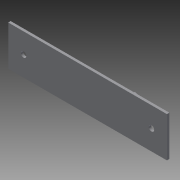
# Autodesk Inventor part: tabliczka tworcy i opiekun boki skrzynki
Saved by Autodesk Inventor 2014 (Build 180170000, 170)
## iProperties
Created: 2018-03-23
Part Number: tabliczka tworcy i opiekun boki skrzynki
Material: Generic
Document SubType Name: Modeling
Designer: HP820
Density: 1 g/cm^3
Appearance: Default
Author: HP820
Autodesk Inventor part; units mm, degrees
(part 1 of 3)
ref_plane "YZ Plane" through (0, 0, 0) normal (1, 0, 0) x (0, 1, 0)
ref_plane "XZ Plane" through (0, 0, 0) normal (0, 1, 0) x (-1, 0, 0)
ref_plane "XY Plane" through (0, 0, 0) normal (0, 0, 1) x (1, 0, 0)
sketch "Sketch1" plane through (0, 0, 0) normal (0, 1, 0) x (-1, 0, 0)
  line L0 (-51.5, 13) -> (51.5, 13)
  line L1 (51.5, 13) -> (51.5, -13)
  line L2 (51.5, -13) -> (-51.5, -13)
  line L3 (-51.5, -13) -> (-51.5, 13)
  line L4 (-51.5, 13) -> (51.5, -13) construction
  line L5 (51.5, 13) -> (-51.5, -13) construction
  point P0 (0, 0)
  dimension "d0" = 103
  dimension "d1" = 26
  constraints: 12 end point, 2 midpoint, 2 parallel, 1 horizontal, 1 perpendicular
  measures "d0" distance of L1.end L2.end
  measures "d1" distance of L0.end L1.end
extrude "Extrusion1" add sketch "Sketch1" along normal blind 1.6
sketch "Sketch2" plane through (0, 1.6, 0) normal (0, 1, 0) x (1, 0, 0)
  line L0 (-48.6354, 11.3005) -> (49.671, 11.3005) construction
  line L1 (49.671, 11.3005) -> (49.671, -11.1656) construction
  line L2 (49.671, -11.1656) -> (-48.6354, -11.1656) construction
  line L3 (-48.6354, -11.1656) -> (-48.6354, 11.3005) construction
  spline S0 degree 2 poles (-15.1532, 10.858) (-15.1532, 10.6489) (-15.2869, 10.2696) (-15.4109, 10.1432) knots 0 0 0 1 2 2 2
  spline S1 degree 2 poles (-15.4109, 10.1432) (-15.4863, 10.063) (-15.671, 9.9317) (-15.7804, 9.8855) knots 0 0 0 1 2 2 2
  spline S2 degree 2 poles (-15.7804, 9.8855) (-15.8923, 9.8393) (-16.1524, 9.7858) (-16.3128, 9.7858) knots 0 0 0 1 2 2 2
  line L4 (-16.3128, 9.7858) -> (-16.7067, 9.7858)
  line L5 (-16.7067, 9.7858) -> (-16.7067, 8.8037)
  line L6 (-16.7067, 8.8037) -> (-17.4603, 8.8037)
  line L7 (-17.4603, 8.8037) -> (-17.4603, 11.8037)
  line L8 (-17.4603, 11.8037) -> (-16.2958, 11.8037)
  spline S3 degree 2 poles (-16.2958, 11.8037) (-16.0381, 11.8037) (-15.6613, 11.7089) (-15.5081, 11.6068) knots 0 0 0 1 2 2 2
  spline S4 degree 2 poles (-15.5081, 11.6068) (-15.338, 11.4925) (-15.1532, 11.1181) (-15.1532, 10.858) knots 0 0 0 1 2 2 2
  spline S5 degree 2 poles (-15.9263, 10.8385) (-15.9263, 10.9674) (-16.0479, 11.1497) (-16.1305, 11.1837) knots 0 0 0 1 2 2 2
  spline S6 degree 2 poles (-16.1305, 11.1837) (-16.2375, 11.2299) (-16.432, 11.2445) (-16.5997, 11.2445) knots 0 0 0 1 2 2 2
  line L9 (-16.5997, 11.2445) -> (-16.7067, 11.2445)
  line L10 (-16.7067, 11.2445) -> (-16.7067, 10.345)
  line L11 (-16.7067, 10.345) -> (-16.6532, 10.345)
  spline S7 degree 2 poles (-16.6532, 10.345) (-16.5487, 10.345) (-16.359, 10.3499) (-16.2885, 10.362) knots 0 0 0 1 2 2 2
  spline S8 degree 2 poles (-16.2885, 10.362) (-16.2278, 10.3717) (-16.094, 10.4301) (-16.0576, 10.4666) knots 0 0 0 1 2 2 2
  spline S9 degree 2 poles (-16.0576, 10.4666) (-15.9798, 10.5395) (-15.9263, 10.7024) (-15.9263, 10.8385) knots 0 0 0 1 2 2 2
  line L12 (-13.2715, 10.3985) -> (-13.3299, 10.3985)
  spline S10 degree 2 poles (-13.3299, 10.3985) (-13.3712, 10.4131) (-13.5244, 10.4277) (-13.6167, 10.4277) knots 0 0 0 1 2 2 2
  spline S11 degree 2 poles (-13.6167, 10.4277) (-13.7261, 10.4277) (-13.9717, 10.362) (-14.0859, 10.3183) knots 0 0 0 1 2 2 2
  line L13 (-14.0859, 10.3183) -> (-14.0859, 8.8037)
  line L14 (-14.0859, 8.8037) -> (-14.791, 8.8037)
  line L15 (-14.791, 8.8037) -> (-14.791, 11.067)
  line L16 (-14.791, 11.067) -> (-14.0859, 11.067)
  line L17 (-14.0859, 11.067) -> (-14.0859, 10.7413)
  spline S12 degree 2 poles (-14.0859, 10.7413) (-14.0373, 10.785) (-13.8671, 10.9212) (-13.7966, 10.9625) knots 0 0 0 1 2 2 2
  spline S13 degree 2 poles (-13.7966, 10.9625) (-13.7188, 11.0087) (-13.5146, 11.0743) (-13.4247, 11.0743) knots 0 0 0 1 2 2 2
  spline S14 degree 2 poles (-13.4247, 11.0743) (-13.3906, 11.0743) (-13.3056, 11.0695) (-13.2715, 11.067) knots 0 0 0 1 2 2 2
  line L18 (-13.2715, 11.067) -> (-13.2715, 10.3985)
  spline S15 degree 2 poles (-10.8307, 9.9341) (-10.8307, 9.375) (-11.4409, 8.7332) (-11.9976, 8.7332) knots 0 0 0 1 2 2 2
  spline S16 degree 2 poles (-11.9976, 8.7332) (-12.5519, 8.7332) (-13.167, 9.375) (-13.167, 9.9341) knots 0 0 0 1 2 2 2
  spline S17 degree 2 poles (-13.167, 9.9341) (-13.167, 10.4982) (-12.5519, 11.1376) (-11.9976, 11.1376) knots 0 0 0 1 2 2 2
  spline S18 degree 2 poles (-11.9976, 11.1376) (-11.4433, 11.1376) (-10.8307, 10.4957) (-10.8307, 9.9341) knots 0 0 0 1 2 2 2
  spline S19 degree 2 poles (-11.5527, 9.9293) (-11.5527, 10.1311) (-11.6184, 10.4009) (-11.6767, 10.4811) knots 0 0 0 1 2 2 2
  spline S20 degree 2 poles (-11.6767, 10.4811) (-11.7399, 10.5662) (-11.8979, 10.6319) (-11.9976, 10.6319) knots 0 0 0 1 2 2 2
  spline S21 degree 2 poles (-11.9976, 10.6319) (-12.0949, 10.6319) (-12.248, 10.5735) (-12.3112, 10.4909) knots 0 0 0 1 2 2 2
  spline S22 degree 2 poles (-12.3112, 10.4909) (-12.372, 10.4131) (-12.4449, 10.1384) (-12.4449, 9.9293) knots 0 0 0 1 2 2 2
  spline S23 degree 2 poles (-12.4449, 9.9293) (-12.4449, 9.7226) (-12.3769, 9.4674) (-12.321, 9.3896) knots 0 0 0 1 2 2 2
  spline S24 degree 2 poles (-12.321, 9.3896) (-12.265, 9.3118) (-12.0949, 9.2388) (-11.9927, 9.2388) knots 0 0 0 1 2 2 2
  spline S25 degree 2 poles (-11.9927, 9.2388) (-11.9077, 9.2388) (-11.7326, 9.3118) (-11.6791, 9.3847) knots 0 0 0 1 2 2 2
  spline S26 degree 2 poles (-11.6791, 9.3847) (-11.6184, 9.4698) (-11.5527, 9.7153) (-11.5527, 9.9293) knots 0 0 0 1 2 2 2
  spline S27 degree 2 poles (-9.4984, 8.7648) (-9.4984, 8.3807) (-9.953, 7.9528) (-10.3128, 7.9528) knots 0 0 0 1 2 2 2
  spline S28 degree 2 poles (-10.3128, 7.9528) (-10.5073, 7.9528) (-10.821, 7.9868) (-10.8939, 8.0063) knots 0 0 0 1 2 2 2
  line L19 (-10.8939, 8.0063) -> (-10.8939, 8.5265)
  line L20 (-10.8939, 8.5265) -> (-10.8404, 8.5265)
  spline S29 degree 2 poles (-10.8404, 8.5265) (-10.7699, 8.5047) (-10.6046, 8.4779) (-10.5535, 8.4779) knots 0 0 0 1 2 2 2
  spline S30 degree 2 poles (-10.5535, 8.4779) (-10.3493, 8.4779) (-10.2034, 8.7283) (-10.2034, 9.0128) knots 0 0 0 1 2 2 2
  line L21 (-10.2034, 9.0128) -> (-10.2034, 10.576)
  line L22 (-10.2034, 10.576) -> (-10.6094, 10.576)
  line L23 (-10.6094, 10.576) -> (-10.6094, 11.067)
  line L24 (-10.6094, 11.067) -> (-9.4984, 11.067)
  line L25 (-9.4984, 11.067) -> (-9.4984, 8.7648)
  line L26 (-9.4984, 11.3904) -> (-10.2496, 11.3904)
  line L27 (-10.2496, 11.3904) -> (-10.2496, 11.9398)
  line L28 (-10.2496, 11.9398) -> (-9.4984, 11.9398)
  line L29 (-9.4984, 11.9398) -> (-9.4984, 11.3904)
  spline S31 degree 2 poles (-7.7991, 8.7429) (-8.4409, 8.7429) (-9.124, 9.3555) (-9.124, 9.922) knots 0 0 0 1 2 2 2
  spline S32 degree 2 poles (-9.124, 9.922) (-9.124, 10.4763) (-8.4871, 11.1376) (-7.9133, 11.1376) knots 0 0 0 1 2 2 2
  spline S33 degree 2 poles (-7.9133, 11.1376) (-7.3955, 11.1376) (-6.8704, 10.576) (-6.8704, 10.0557) knots 0 0 0 1 2 2 2
  line L30 (-6.8704, 10.0557) -> (-6.8704, 9.8004)
  line L31 (-6.8704, 9.8004) -> (-8.419, 9.8004)
  spline S34 degree 2 poles (-8.419, 9.8004) (-8.4093, 9.6424) (-8.295, 9.4333) (-8.2026, 9.3701) knots 0 0 0 1 2 2 2
  spline S35 degree 2 poles (-8.2026, 9.3701) (-8.1127, 9.3069) (-7.8696, 9.2534) (-7.7261, 9.2534) knots 0 0 0 1 2 2 2
  spline S36 degree 2 poles (-7.7261, 9.2534) (-7.6046, 9.2534) (-7.3663, 9.3069) (-7.2667, 9.3531) knots 0 0 0 1 2 2 2
  spline S37 degree 2 poles (-7.2667, 9.3531) (-7.1791, 9.3896) (-7.0333, 9.4795) (-6.9871, 9.5136) knots 0 0 0 1 2 2 2
  line L32 (-6.9871, 9.5136) -> (-6.9117, 9.5136)
  line L33 (-6.9117, 9.5136) -> (-6.9117, 8.9301)
  spline S38 degree 2 poles (-6.9117, 8.9301) (-6.9992, 8.8961) (-7.1402, 8.8377) (-7.2667, 8.8085) knots 0 0 0 1 2 2 2
  spline S39 degree 2 poles (-7.2667, 8.8085) (-7.3809, 8.7769) (-7.624, 8.7429) (-7.7991, 8.7429) knots 0 0 0 1 2 2 2
  spline S40 degree 2 poles (-7.5657, 10.2259) (-7.5705, 10.4495) (-7.7675, 10.6854) (-7.9692, 10.6854) knots 0 0 0 1 2 2 2
  spline S41 degree 2 poles (-7.9692, 10.6854) (-8.1759, 10.6854) (-8.4093, 10.4374) (-8.4214, 10.2259) knots 0 0 0 1 2 2 2
  line L34 (-8.4214, 10.2259) -> (-7.5657, 10.2259)
  line L35 (-4.2423, 8.8037) -> (-5.0811, 8.8037)
  line L36 (-5.0811, 8.8037) -> (-5.6937, 9.7858)
  line L37 (-5.6937, 9.7858) -> (-5.8031, 9.64)
  line L38 (-5.8031, 9.64) -> (-5.8031, 8.8037)
  line L39 (-5.8031, 8.8037) -> (-6.5081, 8.8037)
  line L40 (-6.5081, 8.8037) -> (-6.5081, 11.9374)
  line L41 (-6.5081, 11.9374) -> (-5.8031, 11.9374)
  line L42 (-5.8031, 11.9374) -> (-5.8031, 10.1821)
  line L43 (-5.8031, 10.1821) -> (-5.1346, 11.067)
  line L44 (-5.1346, 11.067) -> (-4.3007, 11.067)
  line L45 (-4.3007, 11.067) -> (-5.0932, 10.0922)
  line L46 (-5.0932, 10.0922) -> (-4.2423, 8.8037)
  spline S42 degree 2 poles (-3.1556, 8.7599) (-3.5859, 8.7599) (-3.9798, 9.1149) (-3.9798, 9.5184) knots 0 0 0 1 2 2 2
  line L47 (-3.9798, 9.5184) -> (-3.9798, 10.576)
  line L48 (-3.9798, 10.576) -> (-4.2496, 10.576)
  line L49 (-4.2496, 10.576) -> (-4.2496, 11.067)
  line L50 (-4.2496, 11.067) -> (-3.9798, 11.067)
  line L51 (-3.9798, 11.067) -> (-3.9798, 11.7137)
  line L52 (-3.9798, 11.7137) -> (-3.2748, 11.7137)
  line L53 (-3.2748, 11.7137) -> (-3.2748, 11.067)
  line L54 (-3.2748, 11.067) -> (-2.594, 11.067)
  line L55 (-2.594, 11.067) -> (-2.594, 10.576)
  line L56 (-2.594, 10.576) -> (-3.2748, 10.576)
  line L57 (-3.2748, 10.576) -> (-3.2748, 9.7713)
  spline S43 degree 2 poles (-3.2748, 9.7713) (-3.2748, 9.6521) (-3.2699, 9.4747) (-3.2407, 9.4042) knots 0 0 0 1 2 2 2
  spline S44 degree 2 poles (-3.2407, 9.4042) (-3.2115, 9.3337) (-3.0681, 9.251) (-2.932, 9.251) knots 0 0 0 1 2 2 2
  spline S45 degree 2 poles (-2.932, 9.251) (-2.8736, 9.251) (-2.6913, 9.2996) (-2.6548, 9.3191) knots 0 0 0 1 2 2 2
  line L58 (-2.6548, 9.3191) -> (-2.594, 9.3191)
  line L59 (-2.594, 9.3191) -> (-2.594, 8.8231)
  spline S46 degree 2 poles (-2.594, 8.8231) (-2.7083, 8.794) (-2.966, 8.7599) (-3.1556, 8.7599) knots 0 0 0 1 2 2 2
  line L60 (2.2731, 11.067) -> (1.6118, 8.8037)
  line L61 (1.6118, 8.8037) -> (0.863, 8.8037)
  line L62 (0.863, 8.8037) -> (0.4643, 10.2672)
  line L63 (0.4643, 10.2672) -> (0.0656, 8.8037)
  line L64 (0.0656, 8.8037) -> (-0.6832, 8.8037)
  line L65 (-0.6832, 8.8037) -> (-1.3396, 11.067)
  line L66 (-1.3396, 11.067) -> (-0.5981, 11.067)
  line L67 (-0.5981, 11.067) -> (-0.2504, 9.5695)
  line L68 (-0.2504, 9.5695) -> (0.1774, 11.067)
  line L69 (0.1774, 11.067) -> (0.8022, 11.067)
  line L70 (0.8022, 11.067) -> (1.2058, 9.5695)
  line L71 (1.2058, 9.5695) -> (1.5486, 11.067)
  line L72 (1.5486, 11.067) -> (2.2731, 11.067)
  line L73 (4.6823, 11.067) -> (3.5421, 7.9747)
  line L74 (3.5421, 7.9747) -> (2.7836, 7.9747)
  line L75 (2.7836, 7.9747) -> (3.1264, 8.8596)
  line L76 (3.1264, 8.8596) -> (2.2974, 11.067)
  line L77 (2.2974, 11.067) -> (3.0364, 11.067)
  line L78 (3.0364, 11.067) -> (3.5129, 9.6473)
  line L79 (3.5129, 9.6473) -> (3.9578, 11.067)
  line L80 (3.9578, 11.067) -> (4.6823, 11.067)
  line L81 (7.2131, 8.8037) -> (6.3744, 8.8037)
  line L82 (6.3744, 8.8037) -> (5.7617, 9.7858)
  line L83 (5.7617, 9.7858) -> (5.6523, 9.64)
  line L84 (5.6523, 9.64) -> (5.6523, 8.8037)
  line L85 (5.6523, 8.8037) -> (4.9473, 8.8037)
  line L86 (4.9473, 8.8037) -> (4.9473, 11.9374)
  line L87 (4.9473, 11.9374) -> (5.6523, 11.9374)
  line L88 (5.6523, 11.9374) -> (5.6523, 10.1821)
  line L89 (5.6523, 10.1821) -> (6.3209, 11.067)
  line L90 (6.3209, 11.067) -> (7.1547, 11.067)
  line L91 (7.1547, 11.067) -> (6.3622, 10.0922)
  line L92 (6.3622, 10.0922) -> (7.2131, 8.8037)
  spline S47 degree 2 poles (9.6053, 9.9341) (9.6053, 9.375) (8.9951, 8.7332) (8.4384, 8.7332) knots 0 0 0 1 2 2 2
  spline S48 degree 2 poles (8.4384, 8.7332) (7.8841, 8.7332) (7.269, 9.375) (7.269, 9.9341) knots 0 0 0 1 2 2 2
  spline S49 degree 2 poles (7.269, 9.9341) (7.269, 10.4982) (7.8841, 11.1376) (8.4384, 11.1376) knots 0 0 0 1 2 2 2
  spline S50 degree 2 poles (8.4384, 11.1376) (8.9927, 11.1376) (9.6053, 10.4957) (9.6053, 9.9341) knots 0 0 0 1 2 2 2
  spline S51 degree 2 poles (8.8833, 9.9293) (8.8833, 10.1311) (8.8176, 10.4009) (8.7593, 10.4811) knots 0 0 0 1 2 2 2
  spline S52 degree 2 poles (8.7593, 10.4811) (8.6961, 10.5662) (8.538, 10.6319) (8.4384, 10.6319) knots 0 0 0 1 2 2 2
  spline S53 degree 2 poles (8.4384, 10.6319) (8.3411, 10.6319) (8.188, 10.5735) (8.1248, 10.4909) knots 0 0 0 1 2 2 2
  spline S54 degree 2 poles (8.1248, 10.4909) (8.064, 10.4131) (7.991, 10.1384) (7.991, 9.9293) knots 0 0 0 1 2 2 2
  spline S55 degree 2 poles (7.991, 9.9293) (7.991, 9.7226) (8.0591, 9.4674) (8.115, 9.3896) knots 0 0 0 1 2 2 2
  spline S56 degree 2 poles (8.115, 9.3896) (8.1709, 9.3118) (8.3411, 9.2388) (8.4432, 9.2388) knots 0 0 0 1 2 2 2
  spline S57 degree 2 poles (8.4432, 9.2388) (8.5283, 9.2388) (8.7034, 9.3118) (8.7568, 9.3847) knots 0 0 0 1 2 2 2
  spline S58 degree 2 poles (8.7568, 9.3847) (8.8176, 9.4698) (8.8833, 9.7153) (8.8833, 9.9293) knots 0 0 0 1 2 2 2
  line L93 (12.0972, 8.8037) -> (11.3873, 8.8037)
  line L94 (11.3873, 8.8037) -> (11.3873, 9.9244)
  spline S59 degree 2 poles (11.3873, 9.9244) (11.3873, 10.063) (11.3654, 10.3353) (11.3363, 10.3985) knots 0 0 0 1 2 2 2
  spline S60 degree 2 poles (11.3363, 10.3985) (11.2998, 10.4763) (11.1637, 10.5419) (11.047, 10.5419) knots 0 0 0 1 2 2 2
  spline S61 degree 2 poles (11.047, 10.5419) (10.9619, 10.5419) (10.7844, 10.4763) (10.6847, 10.4058) knots 0 0 0 1 2 2 2
  line L95 (10.6847, 10.4058) -> (10.6847, 8.8037)
  line L96 (10.6847, 8.8037) -> (9.9797, 8.8037)
  line L97 (9.9797, 8.8037) -> (9.9797, 11.067)
  line L98 (9.9797, 11.067) -> (10.6847, 11.067)
  line L99 (10.6847, 11.067) -> (10.6847, 10.8166)
  spline S62 degree 2 poles (10.6847, 10.8166) (10.8573, 10.9625) (11.1855, 11.1278) (11.3849, 11.1278) knots 0 0 0 1 2 2 2
  spline S63 degree 2 poles (11.3849, 11.1278) (11.7301, 11.1278) (12.0972, 10.6902) (12.0972, 10.2769) knots 0 0 0 1 2 2 2
  line L100 (12.0972, 10.2769) -> (12.0972, 8.8037)
  spline S64 degree 2 poles (13.8671, 9.0444) (13.7941, 8.9836) (13.6799, 8.8863) (13.5826, 8.8377) knots 0 0 0 1 2 2 2
  spline S65 degree 2 poles (13.5826, 8.8377) (13.4878, 8.7915) (13.3079, 8.7429) (13.1474, 8.7429) knots 0 0 0 1 2 2 2
  spline S66 degree 2 poles (13.1474, 8.7429) (12.846, 8.7429) (12.4497, 9.1465) (12.4497, 9.4528) knots 0 0 0 1 2 2 2
  spline S67 degree 2 poles (12.4497, 9.4528) (12.4497, 9.7032) (12.6515, 10.0144) (12.8411, 10.1043) knots 0 0 0 1 2 2 2
  spline S68 degree 2 poles (12.8411, 10.1043) (13.0332, 10.1967) (13.5656, 10.2696) (13.8719, 10.2891) knots 0 0 0 1 2 2 2
  line L101 (13.8719, 10.2891) -> (13.8719, 10.3012)
  spline S69 degree 2 poles (13.8719, 10.3012) (13.8719, 10.4884) (13.5948, 10.6319) (13.3176, 10.6319) knots 0 0 0 1 2 2 2
  spline S70 degree 2 poles (13.3176, 10.6319) (13.1936, 10.6319) (12.8581, 10.5419) (12.7001, 10.4714) knots 0 0 0 1 2 2 2
  line L102 (12.7001, 10.4714) -> (12.6393, 10.4714)
  line L103 (12.6393, 10.4714) -> (12.6393, 11.0184)
  spline S71 degree 2 poles (12.6393, 11.0184) (12.7439, 11.0476) (13.2107, 11.1303) (13.4489, 11.1303) knots 0 0 0 1 2 2 2
  spline S72 degree 2 poles (13.4489, 11.1303) (14.0324, 11.1303) (14.5672, 10.7413) (14.5672, 10.3426) knots 0 0 0 1 2 2 2
  line L104 (14.5672, 10.3426) -> (14.5672, 8.8037)
  line L105 (14.5672, 8.8037) -> (13.8671, 8.8037)
  line L106 (13.8671, 8.8037) -> (13.8671, 9.0444)
  line L107 (13.8671, 9.3944) -> (13.8671, 9.8636)
  spline S73 degree 2 poles (13.8671, 9.8636) (13.6872, 9.8466) (13.4659, 9.8199) (13.359, 9.781) knots 0 0 0 1 2 2 2
  spline S74 degree 2 poles (13.359, 9.781) (13.2641, 9.7494) (13.162, 9.6181) (13.162, 9.5111) knots 0 0 0 1 2 2 2
  spline S75 degree 2 poles (13.162, 9.5111) (13.162, 9.3531) (13.3346, 9.234) (13.5024, 9.234) knots 0 0 0 1 2 2 2
  spline S76 degree 2 poles (13.5024, 9.234) (13.5948, 9.234) (13.7893, 9.3191) (13.8671, 9.3944) knots 0 0 0 1 2 2 2
  line L108 (15.7949, 8.8037) -> (15.0899, 8.8037)
  line L109 (15.0899, 8.8037) -> (15.0899, 11.9374)
  line L110 (15.0899, 11.9374) -> (15.7949, 11.9374)
  line L111 (15.7949, 11.9374) -> (15.7949, 8.8037)
  line L112 (17.0397, 8.8037) -> (16.3346, 8.8037)
  line L113 (16.3346, 8.8037) -> (16.3346, 11.067)
  line L114 (16.3346, 11.067) -> (17.0397, 11.067)
  line L115 (17.0397, 11.067) -> (17.0397, 8.8037)
  line L116 (17.0615, 11.3904) -> (16.3152, 11.3904)
  line L117 (16.3152, 11.3904) -> (16.3152, 11.9398)
  line L118 (16.3152, 11.9398) -> (17.0615, 11.9398)
  line L119 (17.0615, 11.9398) -> (17.0615, 11.3904)
  line L120 (18.4157, 8.8037) -> (17.7034, 8.8037)
  line L121 (17.7034, 8.8037) -> (17.7034, 9.5962)
  line L122 (17.7034, 9.5962) -> (18.4157, 9.5962)
  line L123 (18.4157, 9.5962) -> (18.4157, 8.8037)
  line L124 (18.4157, 10.2745) -> (17.7034, 10.2745)
  line L125 (17.7034, 10.2745) -> (17.7034, 11.067)
  line L126 (17.7034, 11.067) -> (18.4157, 11.067)
  line L127 (18.4157, 11.067) -> (18.4157, 10.2745)
  line L128 (-19.4137, 3.8643) -> (-21.4145, 3.8643)
  line L129 (-21.4145, 3.8643) -> (-21.4145, 4.8173)
  line L130 (-21.4145, 4.8173) -> (-21.7573, 4.613)
  line L131 (-21.7573, 4.613) -> (-21.7573, 5.0968)
  line L132 (-21.7573, 5.0968) -> (-21.4145, 5.2962)
  line L133 (-21.4145, 5.2962) -> (-21.4145, 6.8643)
  line L134 (-21.4145, 6.8643) -> (-20.6658, 6.8643)
  line L135 (-20.6658, 6.8643) -> (-20.6658, 5.7095)
  line L136 (-20.6658, 5.7095) -> (-20.0191, 6.096)
  line L137 (-20.0191, 6.096) -> (-20.0191, 5.6122)
  line L138 (-20.0191, 5.6122) -> (-20.6658, 5.2305)
  line L139 (-20.6658, 5.2305) -> (-20.6658, 4.4356)
  line L140 (-20.6658, 4.4356) -> (-19.4137, 4.4356)
  line L141 (-19.4137, 4.4356) -> (-19.4137, 3.8643)
  line L142 (-16.9948, 3.8643) -> (-17.6998, 3.8643)
  line L143 (-17.6998, 3.8643) -> (-17.6998, 4.1147)
  spline S77 degree 2 poles (-17.6998, 4.1147) (-17.8821, 3.9615) (-18.1885, 3.801) (-18.4, 3.801) knots 0 0 0 1 2 2 2
  spline S78 degree 2 poles (-18.4, 3.801) (-18.7355, 3.801) (-19.1123, 4.2265) (-19.1123, 4.6544) knots 0 0 0 1 2 2 2
  line L144 (-19.1123, 4.6544) -> (-19.1123, 6.1276)
  line L145 (-19.1123, 6.1276) -> (-18.4024, 6.1276)
  line L146 (-18.4024, 6.1276) -> (-18.4024, 5.0045)
  spline S79 degree 2 poles (-18.4024, 5.0045) (-18.4024, 4.8294) (-18.3854, 4.6057) (-18.3513, 4.5304) knots 0 0 0 1 2 2 2
  spline S80 degree 2 poles (-18.3513, 4.5304) (-18.3173, 4.4599) (-18.1836, 4.3869) (-18.062, 4.3869) knots 0 0 0 1 2 2 2
  spline S81 degree 2 poles (-18.062, 4.3869) (-17.9891, 4.3869) (-17.7849, 4.4599) (-17.6998, 4.5231) knots 0 0 0 1 2 2 2
  line L147 (-17.6998, 4.5231) -> (-17.6998, 6.1276)
  line L148 (-17.6998, 6.1276) -> (-16.9948, 6.1276)
  line L149 (-16.9948, 6.1276) -> (-16.9948, 3.8643)
  line L150 (-14.1893, 3.8643) -> (-15.028, 3.8643)
  line L151 (-15.028, 3.8643) -> (-15.6406, 4.8464)
  line L152 (-15.6406, 4.8464) -> (-15.75, 4.7006)
  line L153 (-15.75, 4.7006) -> (-15.75, 3.8643)
  line L154 (-15.75, 3.8643) -> (-16.4551, 3.8643)
  line L155 (-16.4551, 3.8643) -> (-16.4551, 6.998)
  line L156 (-16.4551, 6.998) -> (-15.75, 6.998)
  line L157 (-15.75, 6.998) -> (-15.75, 5.2427)
  line L158 (-15.75, 5.2427) -> (-15.0815, 6.1276)
  line L159 (-15.0815, 6.1276) -> (-14.2476, 6.1276)
  line L160 (-14.2476, 6.1276) -> (-15.0402, 5.1527)
  line L161 (-15.0402, 5.1527) -> (-14.1893, 3.8643)
  spline S82 degree 2 poles (-12.7209, 4.1049) (-12.7938, 4.0442) (-12.9081, 3.9469) (-13.0053, 3.8983) knots 0 0 0 1 2 2 2
  spline S83 degree 2 poles (-13.0053, 3.8983) (-13.1001, 3.8521) (-13.28, 3.8035) (-13.4405, 3.8035) knots 0 0 0 1 2 2 2
  spline S84 degree 2 poles (-13.4405, 3.8035) (-13.7419, 3.8035) (-14.1382, 4.207) (-14.1382, 4.5134) knots 0 0 0 1 2 2 2
  spline S85 degree 2 poles (-14.1382, 4.5134) (-14.1382, 4.7638) (-13.9364, 5.075) (-13.7468, 5.1649) knots 0 0 0 1 2 2 2
  spline S86 degree 2 poles (-13.7468, 5.1649) (-13.5547, 5.2573) (-13.0223, 5.3302) (-12.716, 5.3497) knots 0 0 0 1 2 2 2
  line L162 (-12.716, 5.3497) -> (-12.716, 5.3618)
  spline S87 degree 2 poles (-12.716, 5.3618) (-12.716, 5.549) (-12.9932, 5.6925) (-13.2703, 5.6925) knots 0 0 0 1 2 2 2
  spline S88 degree 2 poles (-13.2703, 5.6925) (-13.3943, 5.6925) (-13.7298, 5.6025) (-13.8878, 5.532) knots 0 0 0 1 2 2 2
  line L163 (-13.8878, 5.532) -> (-13.9486, 5.532)
  line L164 (-13.9486, 5.532) -> (-13.9486, 6.079)
  spline S89 degree 2 poles (-13.9486, 6.079) (-13.844, 6.1082) (-13.3773, 6.1908) (-13.139, 6.1908) knots 0 0 0 1 2 2 2
  spline S90 degree 2 poles (-13.139, 6.1908) (-12.5556, 6.1908) (-12.0207, 5.8019) (-12.0207, 5.4032) knots 0 0 0 1 2 2 2
  line L165 (-12.0207, 5.4032) -> (-12.0207, 3.8643)
  line L166 (-12.0207, 3.8643) -> (-12.7209, 3.8643)
  line L167 (-12.7209, 3.8643) -> (-12.7209, 4.1049)
  line L168 (-12.7209, 4.455) -> (-12.7209, 4.9242)
  spline S91 degree 2 poles (-12.7209, 4.9242) (-12.9008, 4.9072) (-13.122, 4.8805) (-13.229, 4.8416) knots 0 0 0 1 2 2 2
  spline S92 degree 2 poles (-13.229, 4.8416) (-13.3238, 4.81) (-13.4259, 4.6787) (-13.4259, 4.5717) knots 0 0 0 1 2 2 2
  spline S93 degree 2 poles (-13.4259, 4.5717) (-13.4259, 4.4137) (-13.2533, 4.2946) (-13.0855, 4.2946) knots 0 0 0 1 2 2 2
  spline S94 degree 2 poles (-13.0855, 4.2946) (-12.9932, 4.2946) (-12.7987, 4.3797) (-12.7209, 4.455) knots 0 0 0 1 2 2 2
  spline S95 degree 2 poles (-10.81, 3.8035) (-11.058, 3.8035) (-11.5029, 3.9129) (-11.6487, 3.9858) knots 0 0 0 1 2 2 2
  line L169 (-11.6487, 3.9858) -> (-11.6487, 4.5814)
  line L170 (-11.6487, 4.5814) -> (-11.5904, 4.5814)
  spline S96 degree 2 poles (-11.5904, 4.5814) (-11.5393, 4.5425) (-11.4105, 4.4502) (-11.2962, 4.3991) knots 0 0 0 1 2 2 2
  spline S97 degree 2 poles (-11.2962, 4.3991) (-11.1966, 4.3529) (-10.951, 4.2873) (-10.8051, 4.2873) knots 0 0 0 1 2 2 2
  spline S98 degree 2 poles (-10.8051, 4.2873) (-10.6569, 4.2873) (-10.4283, 4.3797) (-10.4283, 4.4793) knots 0 0 0 1 2 2 2
  spline S99 degree 2 poles (-10.4283, 4.4793) (-10.4283, 4.5571) (-10.5329, 4.6398) (-10.6836, 4.6738) knots 0 0 0 1 2 2 2
  spline S100 degree 2 poles (-10.6836, 4.6738) (-10.7638, 4.6957) (-11.0094, 4.7419) (-11.1042, 4.7711) knots 0 0 0 1 2 2 2
  spline S101 degree 2 poles (-11.1042, 4.7711) (-11.3716, 4.8537) (-11.639, 5.1771) (-11.639, 5.4421) knots 0 0 0 1 2 2 2
  spline S102 degree 2 poles (-11.639, 5.4421) (-11.639, 5.5928) (-11.5004, 5.8602) (-11.3643, 5.9647) knots 0 0 0 1 2 2 2
  spline S103 degree 2 poles (-11.3643, 5.9647) (-11.2306, 6.0669) (-10.8343, 6.1884) (-10.5839, 6.1884) knots 0 0 0 1 2 2 2
  spline S104 degree 2 poles (-10.5839, 6.1884) (-10.3457, 6.1884) (-9.947, 6.0936) (-9.8108, 6.028) knots 0 0 0 1 2 2 2
  line L171 (-9.8108, 6.028) -> (-9.8108, 5.4542)
  line L172 (-9.8108, 5.4542) -> (-9.8667, 5.4542)
  spline S105 degree 2 poles (-9.8667, 5.4542) (-9.9032, 5.4834) (-10.0612, 5.5782) (-10.1342, 5.6122) knots 0 0 0 1 2 2 2
  spline S106 degree 2 poles (-10.1342, 5.6122) (-10.2241, 5.6511) (-10.4429, 5.7046) (-10.5572, 5.7046) knots 0 0 0 1 2 2 2
  spline S107 degree 2 poles (-10.5572, 5.7046) (-10.7103, 5.7046) (-10.9218, 5.6001) (-10.9218, 5.515) knots 0 0 0 1 2 2 2
  spline S108 degree 2 poles (-10.9218, 5.515) (-10.9218, 5.4372) (-10.8173, 5.3497) (-10.6423, 5.3059) knots 0 0 0 1 2 2 2
  spline S109 degree 2 poles (-10.6423, 5.3059) (-10.5523, 5.284) (-10.3165, 5.2427) (-10.2071, 5.2062) knots 0 0 0 1 2 2 2
  spline S110 degree 2 poles (-10.2071, 5.2062) (-9.964, 5.1284) (-9.7111, 4.8245) (-9.7111, 4.5717) knots 0 0 0 1 2 2 2
  spline S111 degree 2 poles (-9.7111, 4.5717) (-9.7111, 4.4137) (-9.8594, 4.1244) (-9.998, 4.0271) knots 0 0 0 1 2 2 2
  spline S112 degree 2 poles (-9.998, 4.0271) (-10.1415, 3.9202) (-10.5353, 3.8035) (-10.81, 3.8035) knots 0 0 0 1 2 2 2
  line L173 (-7.5718, 3.8643) -> (-9.5483, 3.8643)
  line L174 (-9.5483, 3.8643) -> (-9.5483, 4.3286)
  line L175 (-9.5483, 4.3286) -> (-8.4688, 5.5976)
  line L176 (-8.4688, 5.5976) -> (-9.4996, 5.5976)
  line L177 (-9.4996, 5.5976) -> (-9.4996, 6.1276)
  line L178 (-9.4996, 6.1276) -> (-7.5936, 6.1276)
  line L179 (-7.5936, 6.1276) -> (-7.5936, 5.6706)
  line L180 (-7.5936, 5.6706) -> (-8.6755, 4.404)
  line L181 (-8.6755, 4.404) -> (-7.5718, 4.404)
  line L182 (-7.5718, 4.404) -> (-7.5718, 3.8643)
  line L183 (-3.3878, 3.8643) -> (-4.1123, 3.8643)
  line L184 (-4.1123, 3.8643) -> (-5.2695, 5.955)
  line L185 (-5.2695, 5.955) -> (-5.2695, 3.8643)
  line L186 (-5.2695, 3.8643) -> (-5.9575, 3.8643)
  line L187 (-5.9575, 3.8643) -> (-5.9575, 6.8643)
  line L188 (-5.9575, 6.8643) -> (-5.0337, 6.8643)
  line L189 (-5.0337, 6.8643) -> (-4.0758, 5.1455)
  line L190 (-4.0758, 5.1455) -> (-4.0758, 6.8643)
  line L191 (-4.0758, 6.8643) -> (-3.3878, 6.8643)
  line L192 (-3.3878, 6.8643) -> (-3.3878, 3.8643)
  spline S113 degree 2 poles (-0.6479, 4.9947) (-0.6479, 4.4356) (-1.2581, 3.7938) (-1.8149, 3.7938) knots 0 0 0 1 2 2 2
  spline S114 degree 2 poles (-1.8149, 3.7938) (-2.3692, 3.7938) (-2.9842, 4.4356) (-2.9842, 4.9947) knots 0 0 0 1 2 2 2
  spline S115 degree 2 poles (-2.9842, 4.9947) (-2.9842, 5.5587) (-2.3692, 6.1981) (-1.8149, 6.1981) knots 0 0 0 1 2 2 2
  spline S116 degree 2 poles (-1.8149, 6.1981) (-1.2606, 6.1981) (-0.6479, 5.5563) (-0.6479, 4.9947) knots 0 0 0 1 2 2 2
  spline S117 degree 2 poles (-1.37, 4.9899) (-1.37, 5.1916) (-1.4356, 5.4615) (-1.494, 5.5417) knots 0 0 0 1 2 2 2
  spline S118 degree 2 poles (-1.494, 5.5417) (-1.5572, 5.6268) (-1.7152, 5.6925) (-1.8149, 5.6925) knots 0 0 0 1 2 2 2
  spline S119 degree 2 poles (-1.8149, 5.6925) (-1.9121, 5.6925) (-2.0653, 5.6341) (-2.1285, 5.5515) knots 0 0 0 1 2 2 2
  spline S120 degree 2 poles (-2.1285, 5.5515) (-2.1893, 5.4737) (-2.2622, 5.1989) (-2.2622, 4.9899) knots 0 0 0 1 2 2 2
  spline S121 degree 2 poles (-2.2622, 4.9899) (-2.2622, 4.7832) (-2.1941, 4.528) (-2.1382, 4.4502) knots 0 0 0 1 2 2 2
  spline S122 degree 2 poles (-2.1382, 4.4502) (-2.0823, 4.3724) (-1.9121, 4.2994) (-1.81, 4.2994) knots 0 0 0 1 2 2 2
  spline S123 degree 2 poles (-1.81, 4.2994) (-1.7249, 4.2994) (-1.5499, 4.3724) (-1.4964, 4.4453) knots 0 0 0 1 2 2 2
  spline S124 degree 2 poles (-1.4964, 4.4453) (-1.4356, 4.5304) (-1.37, 4.7759) (-1.37, 4.9899) knots 0 0 0 1 2 2 2
  line L193 (3.0984, 6.1276) -> (2.4372, 3.8643)
  line L194 (2.4372, 3.8643) -> (1.6884, 3.8643)
  line L195 (1.6884, 3.8643) -> (1.2897, 5.3278)
  line L196 (1.2897, 5.3278) -> (0.891, 3.8643)
  line L197 (0.891, 3.8643) -> (0.1422, 3.8643)
  line L198 (0.1422, 3.8643) -> (-0.5142, 6.1276)
  line L199 (-0.5142, 6.1276) -> (0.2273, 6.1276)
  line L200 (0.2273, 6.1276) -> (0.5749, 4.6301)
  line L201 (0.5749, 4.6301) -> (1.0028, 6.1276)
  line L202 (1.0028, 6.1276) -> (1.6276, 6.1276)
  line L203 (1.6276, 6.1276) -> (2.0312, 4.6301)
  line L204 (2.0312, 4.6301) -> (2.3739, 6.1276)
  line L205 (2.3739, 6.1276) -> (3.0984, 6.1276)
  spline S125 degree 2 poles (4.6446, 4.1049) (4.5717, 4.0442) (4.4574, 3.9469) (4.3602, 3.8983) knots 0 0 0 1 2 2 2
  spline S126 degree 2 poles (4.3602, 3.8983) (4.2654, 3.8521) (4.0855, 3.8035) (3.925, 3.8035) knots 0 0 0 1 2 2 2
  spline S127 degree 2 poles (3.925, 3.8035) (3.6235, 3.8035) (3.2273, 4.207) (3.2273, 4.5134) knots 0 0 0 1 2 2 2
  spline S128 degree 2 poles (3.2273, 4.5134) (3.2273, 4.7638) (3.429, 5.075) (3.6187, 5.1649) knots 0 0 0 1 2 2 2
  spline S129 degree 2 poles (3.6187, 5.1649) (3.8107, 5.2573) (4.3432, 5.3302) (4.6495, 5.3497) knots 0 0 0 1 2 2 2
  line L206 (4.6495, 5.3497) -> (4.6495, 5.3618)
  spline S130 degree 2 poles (4.6495, 5.3618) (4.6495, 5.549) (4.3723, 5.6925) (4.0952, 5.6925) knots 0 0 0 1 2 2 2
  spline S131 degree 2 poles (4.0952, 5.6925) (3.9712, 5.6925) (3.6357, 5.6025) (3.4777, 5.532) knots 0 0 0 1 2 2 2
  line L207 (3.4777, 5.532) -> (3.4169, 5.532)
  line L208 (3.4169, 5.532) -> (3.4169, 6.079)
  spline S132 degree 2 poles (3.4169, 6.079) (3.5214, 6.1082) (3.9882, 6.1908) (4.2265, 6.1908) knots 0 0 0 1 2 2 2
  spline S133 degree 2 poles (4.2265, 6.1908) (4.8099, 6.1908) (5.3448, 5.8019) (5.3448, 5.4032) knots 0 0 0 1 2 2 2
  line L209 (5.3448, 5.4032) -> (5.3448, 3.8643)
  line L210 (5.3448, 3.8643) -> (4.6446, 3.8643)
  line L211 (4.6446, 3.8643) -> (4.6446, 4.1049)
  line L212 (4.6446, 4.455) -> (4.6446, 4.9242)
  spline S134 degree 2 poles (4.6446, 4.9242) (4.4647, 4.9072) (4.2435, 4.8805) (4.1365, 4.8416) knots 0 0 0 1 2 2 2
  spline S135 degree 2 poles (4.1365, 4.8416) (4.0417, 4.81) (3.9396, 4.6787) (3.9396, 4.5717) knots 0 0 0 1 2 2 2
  spline S136 degree 2 poles (3.9396, 4.5717) (3.9396, 4.4137) (4.1122, 4.2946) (4.2799, 4.2946) knots 0 0 0 1 2 2 2
  spline S137 degree 2 poles (4.2799, 4.2946) (4.3723, 4.2946) (4.5668, 4.3797) (4.6446, 4.455) knots 0 0 0 1 2 2 2
  line L213 (7.3869, 5.4591) -> (7.3286, 5.4591)
  spline S138 degree 2 poles (7.3286, 5.4591) (7.2872, 5.4737) (7.1341, 5.4882) (7.0417, 5.4882) knots 0 0 0 1 2 2 2
  spline S139 degree 2 poles (7.0417, 5.4882) (6.9323, 5.4882) (6.6867, 5.4226) (6.5725, 5.3788) knots 0 0 0 1 2 2 2
  line L214 (6.5725, 5.3788) -> (6.5725, 3.8643)
  line L215 (6.5725, 3.8643) -> (5.8675, 3.8643)
  line L216 (5.8675, 3.8643) -> (5.8675, 6.1276)
  line L217 (5.8675, 6.1276) -> (6.5725, 6.1276)
  line L218 (6.5725, 6.1276) -> (6.5725, 5.8019)
  spline S140 degree 2 poles (6.5725, 5.8019) (6.6211, 5.8456) (6.7913, 5.9818) (6.8618, 6.0231) knots 0 0 0 1 2 2 2
  spline S141 degree 2 poles (6.8618, 6.0231) (6.9396, 6.0693) (7.1438, 6.1349) (7.2337, 6.1349) knots 0 0 0 1 2 2 2
  spline S142 degree 2 poles (7.2337, 6.1349) (7.2678, 6.1349) (7.3529, 6.1301) (7.3869, 6.1276) knots 0 0 0 1 2 2 2
  line L219 (7.3869, 6.1276) -> (7.3869, 5.4591)
  line L220 (9.9226, 3.8643) -> (9.0838, 3.8643)
  line L221 (9.0838, 3.8643) -> (8.4712, 4.8464)
  line L222 (8.4712, 4.8464) -> (8.3618, 4.7006)
  line L223 (8.3618, 4.7006) -> (8.3618, 3.8643)
  line L224 (8.3618, 3.8643) -> (7.6568, 3.8643)
  line L225 (7.6568, 3.8643) -> (7.6568, 6.998)
  line L226 (7.6568, 6.998) -> (8.3618, 6.998)
  line L227 (8.3618, 6.998) -> (8.3618, 5.2427)
  line L228 (8.3618, 5.2427) -> (9.0303, 6.1276)
  line L229 (9.0303, 6.1276) -> (9.8642, 6.1276)
  line L230 (9.8642, 6.1276) -> (9.0717, 5.1527)
  line L231 (9.0717, 5.1527) -> (9.9226, 3.8643)
  line L232 (10.8488, 3.8643) -> (10.1438, 3.8643)
  line L233 (10.1438, 3.8643) -> (10.1438, 6.1276)
  line L234 (10.1438, 6.1276) -> (10.8488, 6.1276)
  line L235 (10.8488, 6.1276) -> (10.8488, 3.8643)
  line L236 (10.8707, 6.451) -> (10.1243, 6.451)
  line L237 (10.1243, 6.451) -> (10.1243, 7.0004)
  line L238 (10.1243, 7.0004) -> (10.8707, 7.0004)
  line L239 (10.8707, 7.0004) -> (10.8707, 6.451)
  spline S143 degree 2 poles (12.5482, 3.8035) (11.9064, 3.8035) (11.2232, 4.4161) (11.2232, 4.9826) knots 0 0 0 1 2 2 2
  spline S144 degree 2 poles (11.2232, 4.9826) (11.2232, 5.5369) (11.8602, 6.1981) (12.4339, 6.1981) knots 0 0 0 1 2 2 2
  spline S145 degree 2 poles (12.4339, 6.1981) (12.9517, 6.1981) (13.4769, 5.6365) (13.4769, 5.1163) knots 0 0 0 1 2 2 2
  line L240 (13.4769, 5.1163) -> (13.4769, 4.861)
  line L241 (13.4769, 4.861) -> (11.9282, 4.861)
  spline S146 degree 2 poles (11.9282, 4.861) (11.938, 4.703) (12.0522, 4.4939) (12.1446, 4.4307) knots 0 0 0 1 2 2 2
  spline S147 degree 2 poles (12.1446, 4.4307) (12.2346, 4.3675) (12.4777, 4.314) (12.6211, 4.314) knots 0 0 0 1 2 2 2
  spline S148 degree 2 poles (12.6211, 4.314) (12.7427, 4.314) (12.9809, 4.3675) (13.0806, 4.4137) knots 0 0 0 1 2 2 2
  spline S149 degree 2 poles (13.0806, 4.4137) (13.1681, 4.4502) (13.314, 4.5401) (13.3602, 4.5741) knots 0 0 0 1 2 2 2
  line L242 (13.3602, 4.5741) -> (13.4355, 4.5741)
  line L243 (13.4355, 4.5741) -> (13.4355, 3.9907)
  spline S150 degree 2 poles (13.4355, 3.9907) (13.348, 3.9566) (13.207, 3.8983) (13.0806, 3.8691) knots 0 0 0 1 2 2 2
  spline S151 degree 2 poles (13.0806, 3.8691) (12.9663, 3.8375) (12.7232, 3.8035) (12.5482, 3.8035) knots 0 0 0 1 2 2 2
  spline S152 degree 2 poles (12.7816, 5.2865) (12.7767, 5.5101) (12.5798, 5.7459) (12.378, 5.7459) knots 0 0 0 1 2 2 2
  spline S153 degree 2 poles (12.378, 5.7459) (12.1714, 5.7459) (11.938, 5.498) (11.9258, 5.2865) knots 0 0 0 1 2 2 2
  line L244 (11.9258, 5.2865) -> (12.7816, 5.2865)
  line L245 (17.2111, 6.1276) -> (16.5498, 3.8643)
  line L246 (16.5498, 3.8643) -> (15.801, 3.8643)
  line L247 (15.801, 3.8643) -> (15.4023, 5.3278)
  line L248 (15.4023, 5.3278) -> (15.0036, 3.8643)
  line L249 (15.0036, 3.8643) -> (14.2548, 3.8643)
  line L250 (14.2548, 3.8643) -> (13.5984, 6.1276)
  line L251 (13.5984, 6.1276) -> (14.3399, 6.1276)
  line L252 (14.3399, 6.1276) -> (14.6876, 4.6301)
  line L253 (14.6876, 4.6301) -> (15.1154, 6.1276)
  line L254 (15.1154, 6.1276) -> (15.7402, 6.1276)
  line L255 (15.7402, 6.1276) -> (16.1438, 4.6301)
  line L256 (16.1438, 4.6301) -> (16.4866, 6.1276)
  line L257 (16.4866, 6.1276) -> (17.2111, 6.1276)
  line L258 (18.2151, 3.8643) -> (17.5101, 3.8643)
  line L259 (17.5101, 3.8643) -> (17.5101, 6.1276)
  line L260 (17.5101, 6.1276) -> (18.2151, 6.1276)
  line L261 (18.2151, 6.1276) -> (18.2151, 3.8643)
  line L262 (18.237, 6.451) -> (17.4906, 6.451)
  line L263 (17.4906, 6.451) -> (17.4906, 7.0004)
  line L264 (17.4906, 7.0004) -> (18.237, 7.0004)
  line L265 (18.237, 7.0004) -> (18.237, 6.451)
  spline S154 degree 2 poles (19.8634, 3.8035) (19.5838, 3.8035) (19.1195, 3.9445) (18.9469, 4.0904) knots 0 0 0 1 2 2 2
  spline S155 degree 2 poles (18.9469, 4.0904) (18.7791, 4.2386) (18.5895, 4.6835) (18.5895, 4.985) knots 0 0 0 1 2 2 2
  spline S156 degree 2 poles (18.5895, 4.985) (18.5895, 5.3108) (18.7937, 5.7654) (18.9712, 5.9113) knots 0 0 0 1 2 2 2
  spline S157 degree 2 poles (18.9712, 5.9113) (19.1389, 6.0523) (19.596, 6.1884) (19.844, 6.1884) knots 0 0 0 1 2 2 2
  spline S158 degree 2 poles (19.844, 6.1884) (20.0312, 6.1884) (20.4055, 6.1009) (20.5952, 6.0061) knots 0 0 0 1 2 2 2
  line L266 (20.5952, 6.0061) -> (20.5952, 5.4032)
  line L267 (20.5952, 5.4032) -> (20.5052, 5.4032)
  spline S159 degree 2 poles (20.5052, 5.4032) (20.4615, 5.4445) (20.3399, 5.5417) (20.267, 5.5806) knots 0 0 0 1 2 2 2
  spline S160 degree 2 poles (20.267, 5.5806) (20.1892, 5.6244) (19.9971, 5.6827) (19.878, 5.6827) knots 0 0 0 1 2 2 2
  spline S161 degree 2 poles (19.878, 5.6827) (19.6081, 5.6827) (19.3115, 5.3059) (19.3115, 4.985) knots 0 0 0 1 2 2 2
  spline S162 degree 2 poles (19.3115, 4.985) (19.3115, 4.6446) (19.6276, 4.3092) (19.8902, 4.3092) knots 0 0 0 1 2 2 2
  spline S163 degree 2 poles (19.8902, 4.3092) (20.0239, 4.3092) (20.2232, 4.3699) (20.2961, 4.4137) knots 0 0 0 1 2 2 2
  spline S164 degree 2 poles (20.2961, 4.4137) (20.3667, 4.455) (20.4688, 4.5474) (20.5052, 4.5839) knots 0 0 0 1 2 2 2
  line L268 (20.5052, 4.5839) -> (20.5952, 4.5839)
  line L269 (20.5952, 4.5839) -> (20.5952, 3.9785)
  spline S165 degree 2 poles (20.5952, 3.9785) (20.5344, 3.9518) (20.3764, 3.8837) (20.2937, 3.8618) knots 0 0 0 1 2 2 2
  spline S166 degree 2 poles (20.2937, 3.8618) (20.1916, 3.8327) (20.0117, 3.8035) (19.8634, 3.8035) knots 0 0 0 1 2 2 2
  line L270 (22.7346, 3.8643) -> (20.7581, 3.8643)
  line L271 (20.7581, 3.8643) -> (20.7581, 4.3286)
  line L272 (20.7581, 4.3286) -> (21.8375, 5.5976)
  line L273 (21.8375, 5.5976) -> (20.8067, 5.5976)
  line L274 (20.8067, 5.5976) -> (20.8067, 6.1276)
  line L275 (20.8067, 6.1276) -> (22.7127, 6.1276)
  line L276 (22.7127, 6.1276) -> (22.7127, 5.6706)
  line L277 (22.7127, 5.6706) -> (21.6308, 4.404)
  line L278 (21.6308, 4.404) -> (22.7346, 4.404)
  line L279 (22.7346, 4.404) -> (22.7346, 3.8643)
  spline S167 degree 2 poles (-14.5564, -0.1951) (-14.5564, -0.3896) (-14.6901, -0.7348) (-14.8238, -0.8564) knots 0 0 0 1 2 2 2
  spline S168 degree 2 poles (-14.8238, -0.8564) (-14.9745, -0.9925) (-15.3854, -1.1214) (-15.6528, -1.1214) knots 0 0 0 1 2 2 2
  spline S169 degree 2 poles (-15.6528, -1.1214) (-15.8522, -1.1214) (-16.2022, -1.0922) (-16.3359, -1.063) knots 0 0 0 1 2 2 2
  line L280 (-16.3359, -1.063) -> (-16.3359, -0.4552)
  line L281 (-16.3359, -0.4552) -> (-16.2679, -0.4552)
  spline S170 degree 2 poles (-16.2679, -0.4552) (-16.1779, -0.4917) (-15.981, -0.5549) (-15.8254, -0.5549) knots 0 0 0 1 2 2 2
  spline S171 degree 2 poles (-15.8254, -0.5549) (-15.6261, -0.5549) (-15.4097, -0.4431) (-15.3659, -0.341) knots 0 0 0 1 2 2 2
  spline S172 degree 2 poles (-15.3659, -0.341) (-15.3197, -0.2413) (-15.31, 0.0164) (-15.31, 0.1769) knots 0 0 0 1 2 2 2
  line L282 (-15.31, 0.1769) -> (-15.31, 1.3803)
  line L283 (-15.31, 1.3803) -> (-15.9956, 1.3803)
  line L284 (-15.9956, 1.3803) -> (-15.9956, 1.9248)
  line L285 (-15.9956, 1.9248) -> (-14.5564, 1.9248)
  line L286 (-14.5564, 1.9248) -> (-14.5564, -0.1951)
  spline S173 degree 2 poles (-12.7671, -0.8345) (-12.84, -0.8953) (-12.9543, -0.9925) (-13.0515, -1.0411) knots 0 0 0 1 2 2 2
  spline S174 degree 2 poles (-13.0515, -1.0411) (-13.1463, -1.0873) (-13.3262, -1.1359) (-13.4867, -1.1359) knots 0 0 0 1 2 2 2
  spline S175 degree 2 poles (-13.4867, -1.1359) (-13.7881, -1.1359) (-14.1844, -0.7324) (-14.1844, -0.4261) knots 0 0 0 1 2 2 2
  spline S176 degree 2 poles (-14.1844, -0.4261) (-14.1844, -0.1757) (-13.9826, 0.1355) (-13.793, 0.2255) knots 0 0 0 1 2 2 2
  spline S177 degree 2 poles (-13.793, 0.2255) (-13.6009, 0.3179) (-13.0685, 0.3908) (-12.7622, 0.4102) knots 0 0 0 1 2 2 2
  line L287 (-12.7622, 0.4102) -> (-12.7622, 0.4224)
  spline S178 degree 2 poles (-12.7622, 0.4224) (-12.7622, 0.6096) (-13.0393, 0.753) (-13.3165, 0.753) knots 0 0 0 1 2 2 2
  spline S179 degree 2 poles (-13.3165, 0.753) (-13.4405, 0.753) (-13.776, 0.6631) (-13.934, 0.5926) knots 0 0 0 1 2 2 2
  line L288 (-13.934, 0.5926) -> (-13.9948, 0.5926)
  line L289 (-13.9948, 0.5926) -> (-13.9948, 1.1396)
  spline S180 degree 2 poles (-13.9948, 1.1396) (-13.8902, 1.1688) (-13.4235, 1.2514) (-13.1852, 1.2514) knots 0 0 0 1 2 2 2
  spline S181 degree 2 poles (-13.1852, 1.2514) (-12.6017, 1.2514) (-12.0669, 0.8624) (-12.0669, 0.4637) knots 0 0 0 1 2 2 2
  line L290 (-12.0669, 0.4637) -> (-12.0669, -1.0752)
  line L291 (-12.0669, -1.0752) -> (-12.7671, -1.0752)
  line L292 (-12.7671, -1.0752) -> (-12.7671, -0.8345)
  line L293 (-12.7671, -0.4844) -> (-12.7671, -0.0152)
  spline S182 degree 2 poles (-12.7671, -0.0152) (-12.947, -0.0322) (-13.1682, -0.059) (-13.2752, -0.0979) knots 0 0 0 1 2 2 2
  spline S183 degree 2 poles (-13.2752, -0.0979) (-13.37, -0.1295) (-13.4721, -0.2607) (-13.4721, -0.3677) knots 0 0 0 1 2 2 2
  spline S184 degree 2 poles (-13.4721, -0.3677) (-13.4721, -0.5257) (-13.2995, -0.6449) (-13.1317, -0.6449) knots 0 0 0 1 2 2 2
  spline S185 degree 2 poles (-13.1317, -0.6449) (-13.0393, -0.6449) (-12.8449, -0.5598) (-12.7671, -0.4844) knots 0 0 0 1 2 2 2
  spline S186 degree 2 poles (-10.4356, -1.1359) (-10.7152, -1.1359) (-11.1795, -0.9949) (-11.3521, -0.8491) knots 0 0 0 1 2 2 2
  spline S187 degree 2 poles (-11.3521, -0.8491) (-11.5199, -0.7008) (-11.7095, -0.2559) (-11.7095, 0.0456) knots 0 0 0 1 2 2 2
  spline S188 degree 2 poles (-11.7095, 0.0456) (-11.7095, 0.3714) (-11.5053, 0.826) (-11.3278, 0.9718) knots 0 0 0 1 2 2 2
  spline S189 degree 2 poles (-11.3278, 0.9718) (-11.1601, 1.1128) (-10.703, 1.249) (-10.4551, 1.249) knots 0 0 0 1 2 2 2
  spline S190 degree 2 poles (-10.4551, 1.249) (-10.2679, 1.249) (-9.8935, 1.1615) (-9.7039, 1.0667) knots 0 0 0 1 2 2 2
  line L294 (-9.7039, 1.0667) -> (-9.7039, 0.4637)
  line L295 (-9.7039, 0.4637) -> (-9.7938, 0.4637)
  spline S191 degree 2 poles (-9.7938, 0.4637) (-9.8376, 0.5051) (-9.9591, 0.6023) (-10.0321, 0.6412) knots 0 0 0 1 2 2 2
  spline S192 degree 2 poles (-10.0321, 0.6412) (-10.1098, 0.685) (-10.3019, 0.7433) (-10.421, 0.7433) knots 0 0 0 1 2 2 2
  spline S193 degree 2 poles (-10.421, 0.7433) (-10.6909, 0.7433) (-10.9875, 0.3665) (-10.9875, 0.0456) knots 0 0 0 1 2 2 2
  spline S194 degree 2 poles (-10.9875, 0.0456) (-10.9875, -0.2948) (-10.6714, -0.6303) (-10.4089, -0.6303) knots 0 0 0 1 2 2 2
  spline S195 degree 2 poles (-10.4089, -0.6303) (-10.2752, -0.6303) (-10.0758, -0.5695) (-10.0029, -0.5257) knots 0 0 0 1 2 2 2
  spline S196 degree 2 poles (-10.0029, -0.5257) (-9.9324, -0.4844) (-9.8303, -0.392) (-9.7938, -0.3556) knots 0 0 0 1 2 2 2
  line L296 (-9.7938, -0.3556) -> (-9.7039, -0.3556)
  line L297 (-9.7039, -0.3556) -> (-9.7039, -0.9609)
  spline S197 degree 2 poles (-9.7039, -0.9609) (-9.7646, -0.9876) (-9.9227, -1.0557) (-10.0053, -1.0776) knots 0 0 0 1 2 2 2
  spline S198 degree 2 poles (-10.0053, -1.0776) (-10.1074, -1.1068) (-10.2873, -1.1359) (-10.4356, -1.1359) knots 0 0 0 1 2 2 2
  spline S199 degree 2 poles (-8.2087, -1.1359) (-8.8505, -1.1359) (-9.5337, -0.5233) (-9.5337, 0.0432) knots 0 0 0 1 2 2 2
  spline S200 degree 2 poles (-9.5337, 0.0432) (-9.5337, 0.5974) (-8.8967, 1.2587) (-8.323, 1.2587) knots 0 0 0 1 2 2 2
  spline S201 degree 2 poles (-8.323, 1.2587) (-7.8051, 1.2587) (-7.28, 0.6971) (-7.28, 0.1769) knots 0 0 0 1 2 2 2
  line L298 (-7.28, 0.1769) -> (-7.28, -0.0784)
  line L299 (-7.28, -0.0784) -> (-8.8286, -0.0784)
  spline S202 degree 2 poles (-8.8286, -0.0784) (-8.8189, -0.2364) (-8.7047, -0.4455) (-8.6123, -0.5087) knots 0 0 0 1 2 2 2
  spline S203 degree 2 poles (-8.6123, -0.5087) (-8.5223, -0.5719) (-8.2792, -0.6254) (-8.1358, -0.6254) knots 0 0 0 1 2 2 2
  spline S204 degree 2 poles (-8.1358, -0.6254) (-8.0142, -0.6254) (-7.776, -0.5719) (-7.6763, -0.5257) knots 0 0 0 1 2 2 2
  spline S205 degree 2 poles (-7.6763, -0.5257) (-7.5888, -0.4893) (-7.4429, -0.3993) (-7.3967, -0.3653) knots 0 0 0 1 2 2 2
  line L300 (-7.3967, -0.3653) -> (-7.3214, -0.3653)
  line L301 (-7.3214, -0.3653) -> (-7.3214, -0.9487)
  spline S206 degree 2 poles (-7.3214, -0.9487) (-7.4089, -0.9828) (-7.5499, -1.0411) (-7.6763, -1.0703) knots 0 0 0 1 2 2 2
  spline S207 degree 2 poles (-7.6763, -1.0703) (-7.7906, -1.1019) (-8.0337, -1.1359) (-8.2087, -1.1359) knots 0 0 0 1 2 2 2
  spline S208 degree 2 poles (-7.9753, 0.347) (-7.9802, 0.5707) (-8.1771, 0.8065) (-8.3789, 0.8065) knots 0 0 0 1 2 2 2
  spline S209 degree 2 poles (-8.3789, 0.8065) (-8.5855, 0.8065) (-8.8189, 0.5585) (-8.8311, 0.347) knots 0 0 0 1 2 2 2
  line L302 (-8.8311, 0.347) -> (-7.9753, 0.347)
  line L303 (-4.652, -1.0752) -> (-5.4907, -1.0752)
  line L304 (-5.4907, -1.0752) -> (-6.1034, -0.093)
  line L305 (-6.1034, -0.093) -> (-6.2128, -0.2389)
  line L306 (-6.2128, -0.2389) -> (-6.2128, -1.0752)
  line L307 (-6.2128, -1.0752) -> (-6.9178, -1.0752)
  line L308 (-6.9178, -1.0752) -> (-6.9178, 2.0585)
  line L309 (-6.9178, 2.0585) -> (-6.2128, 2.0585)
  line L310 (-6.2128, 2.0585) -> (-6.2128, 0.3033)
  line L311 (-6.2128, 0.3033) -> (-5.5442, 1.1882)
  line L312 (-5.5442, 1.1882) -> (-4.7103, 1.1882)
  line L313 (-4.7103, 1.1882) -> (-5.5029, 0.2133)
  line L314 (-5.5029, 0.2133) -> (-4.652, -1.0752)
  line L315 (-0.118, -1.0752) -> (-0.8667, -1.0752)
  line L316 (-0.8667, -1.0752) -> (-0.8667, 0.9135)
  line L317 (-0.8667, 0.9135) -> (-1.4113, -0.3701)
  line L318 (-1.4113, -0.3701) -> (-1.9267, -0.3701)
  line L319 (-1.9267, -0.3701) -> (-2.4713, 0.9135)
  line L320 (-2.4713, 0.9135) -> (-2.4713, -1.0752)
  line L321 (-2.4713, -1.0752) -> (-3.1812, -1.0752)
  line L322 (-3.1812, -1.0752) -> (-3.1812, 1.9248)
  line L323 (-3.1812, 1.9248) -> (-2.3133, 1.9248)
  line L324 (-2.3133, 1.9248) -> (-1.6471, 0.4443)
  line L325 (-1.6471, 0.4443) -> (-0.9859, 1.9248)
  line L326 (-0.9859, 1.9248) -> (-0.118, 1.9248)
  line L327 (-0.118, 1.9248) -> (-0.118, -1.0752)
  spline S210 degree 2 poles (1.7102, -0.8345) (1.6373, -0.8953) (1.5231, -0.9925) (1.4258, -1.0411) knots 0 0 0 1 2 2 2
  spline S211 degree 2 poles (1.4258, -1.0411) (1.331, -1.0873) (1.1511, -1.1359) (0.9906, -1.1359) knots 0 0 0 1 2 2 2
  spline S212 degree 2 poles (0.9906, -1.1359) (0.6892, -1.1359) (0.2929, -0.7324) (0.2929, -0.4261) knots 0 0 0 1 2 2 2
  spline S213 degree 2 poles (0.2929, -0.4261) (0.2929, -0.1757) (0.4947, 0.1355) (0.6843, 0.2255) knots 0 0 0 1 2 2 2
  spline S214 degree 2 poles (0.6843, 0.2255) (0.8764, 0.3179) (1.4088, 0.3908) (1.7151, 0.4102) knots 0 0 0 1 2 2 2
  line L328 (1.7151, 0.4102) -> (1.7151, 0.4224)
  spline S215 degree 2 poles (1.7151, 0.4224) (1.7151, 0.6096) (1.438, 0.753) (1.1608, 0.753) knots 0 0 0 1 2 2 2
  spline S216 degree 2 poles (1.1608, 0.753) (1.0368, 0.753) (0.7013, 0.6631) (0.5433, 0.5926) knots 0 0 0 1 2 2 2
  line L329 (0.5433, 0.5926) -> (0.4825, 0.5926)
  line L330 (0.4825, 0.5926) -> (0.4825, 1.1396)
  spline S217 degree 2 poles (0.4825, 1.1396) (0.5871, 1.1688) (1.0538, 1.2514) (1.2921, 1.2514) knots 0 0 0 1 2 2 2
  spline S218 degree 2 poles (1.2921, 1.2514) (1.8756, 1.2514) (2.4104, 0.8624) (2.4104, 0.4637) knots 0 0 0 1 2 2 2
  line L331 (2.4104, 0.4637) -> (2.4104, -1.0752)
  line L332 (2.4104, -1.0752) -> (1.7102, -1.0752)
  line L333 (1.7102, -1.0752) -> (1.7102, -0.8345)
  line L334 (1.7102, -0.4844) -> (1.7102, -0.0152)
  spline S219 degree 2 poles (1.7102, -0.0152) (1.5303, -0.0322) (1.3091, -0.059) (1.2021, -0.0979) knots 0 0 0 1 2 2 2
  spline S220 degree 2 poles (1.2021, -0.0979) (1.1073, -0.1295) (1.0052, -0.2607) (1.0052, -0.3677) knots 0 0 0 1 2 2 2
  spline S221 degree 2 poles (1.0052, -0.3677) (1.0052, -0.5257) (1.1778, -0.6449) (1.3456, -0.6449) knots 0 0 0 1 2 2 2
  spline S222 degree 2 poles (1.3456, -0.6449) (1.438, -0.6449) (1.6325, -0.5598) (1.7102, -0.4844) knots 0 0 0 1 2 2 2
  line L335 (4.4526, 0.5196) -> (4.3942, 0.5196)
  spline S223 degree 2 poles (4.3942, 0.5196) (4.3529, 0.5342) (4.1997, 0.5488) (4.1073, 0.5488) knots 0 0 0 1 2 2 2
  spline S224 degree 2 poles (4.1073, 0.5488) (3.9979, 0.5488) (3.7524, 0.4832) (3.6381, 0.4394) knots 0 0 0 1 2 2 2
  line L336 (3.6381, 0.4394) -> (3.6381, -1.0752)
  line L337 (3.6381, -1.0752) -> (2.9331, -1.0752)
  line L338 (2.9331, -1.0752) -> (2.9331, 1.1882)
  line L339 (2.9331, 1.1882) -> (3.6381, 1.1882)
  line L340 (3.6381, 1.1882) -> (3.6381, 0.8624)
  spline S225 degree 2 poles (3.6381, 0.8624) (3.6867, 0.9062) (3.8569, 1.0423) (3.9274, 1.0837) knots 0 0 0 1 2 2 2
  spline S226 degree 2 poles (3.9274, 1.0837) (4.0052, 1.1299) (4.2094, 1.1955) (4.2994, 1.1955) knots 0 0 0 1 2 2 2
  spline S227 degree 2 poles (4.2994, 1.1955) (4.3334, 1.1955) (4.4185, 1.1906) (4.4526, 1.1882) knots 0 0 0 1 2 2 2
  line L341 (4.4526, 1.1882) -> (4.4526, 0.5196)
  spline S228 degree 2 poles (5.5879, -1.1189) (5.1576, -1.1189) (4.7637, -0.764) (4.7637, -0.3604) knots 0 0 0 1 2 2 2
  line L342 (4.7637, -0.3604) -> (4.7637, 0.6971)
  line L343 (4.7637, 0.6971) -> (4.4939, 0.6971)
  line L344 (4.4939, 0.6971) -> (4.4939, 1.1882)
  line L345 (4.4939, 1.1882) -> (4.7637, 1.1882)
  line L346 (4.7637, 1.1882) -> (4.7637, 1.8349)
  line L347 (4.7637, 1.8349) -> (5.4688, 1.8349)
  line L348 (5.4688, 1.8349) -> (5.4688, 1.1882)
  line L349 (5.4688, 1.1882) -> (6.1495, 1.1882)
  line L350 (6.1495, 1.1882) -> (6.1495, 0.6971)
  line L351 (6.1495, 0.6971) -> (5.4688, 0.6971)
  line L352 (5.4688, 0.6971) -> (5.4688, -0.1076)
  spline S229 degree 2 poles (5.4688, -0.1076) (5.4688, -0.2267) (5.4736, -0.4042) (5.5028, -0.4747) knots 0 0 0 1 2 2 2
  spline S230 degree 2 poles (5.5028, -0.4747) (5.532, -0.5452) (5.6754, -0.6278) (5.8115, -0.6278) knots 0 0 0 1 2 2 2
  spline S231 degree 2 poles (5.8115, -0.6278) (5.8699, -0.6278) (6.0522, -0.5792) (6.0887, -0.5598) knots 0 0 0 1 2 2 2
  line L353 (6.0887, -0.5598) -> (6.1495, -0.5598)
  line L354 (6.1495, -0.5598) -> (6.1495, -1.0557)
  spline S232 degree 2 poles (6.1495, -1.0557) (6.0352, -1.0849) (5.7775, -1.1189) (5.5879, -1.1189) knots 0 0 0 1 2 2 2
  line L355 (8.5466, 1.1882) -> (7.4064, -1.9042)
  line L356 (7.4064, -1.9042) -> (6.6479, -1.9042)
  line L357 (6.6479, -1.9042) -> (6.9906, -1.0192)
  line L358 (6.9906, -1.0192) -> (6.1616, 1.1882)
  line L359 (6.1616, 1.1882) -> (6.9007, 1.1882)
  line L360 (6.9007, 1.1882) -> (7.3772, -0.2316)
  line L361 (7.3772, -0.2316) -> (7.8221, 1.1882)
  line L362 (7.8221, 1.1882) -> (8.5466, 1.1882)
  line L363 (10.9291, -1.0752) -> (10.2192, -1.0752)
  line L364 (10.2192, -1.0752) -> (10.2192, 0.0456)
  spline S233 degree 2 poles (10.2192, 0.0456) (10.2192, 0.1842) (10.1973, 0.4564) (10.1681, 0.5196) knots 0 0 0 1 2 2 2
  spline S234 degree 2 poles (10.1681, 0.5196) (10.1316, 0.5974) (9.9955, 0.6631) (9.8788, 0.6631) knots 0 0 0 1 2 2 2
  spline S235 degree 2 poles (9.8788, 0.6631) (9.7937, 0.6631) (9.6162, 0.5974) (9.5166, 0.5269) knots 0 0 0 1 2 2 2
  line L365 (9.5166, 0.5269) -> (9.5166, -1.0752)
  line L366 (9.5166, -1.0752) -> (8.8115, -1.0752)
  line L367 (8.8115, -1.0752) -> (8.8115, 1.1882)
  line L368 (8.8115, 1.1882) -> (9.5166, 1.1882)
  line L369 (9.5166, 1.1882) -> (9.5166, 0.9378)
  spline S236 degree 2 poles (9.5166, 0.9378) (9.6892, 1.0837) (10.0174, 1.249) (10.2167, 1.249) knots 0 0 0 1 2 2 2
  spline S237 degree 2 poles (10.2167, 1.249) (10.562, 1.249) (10.9291, 0.8114) (10.9291, 0.3981) knots 0 0 0 1 2 2 2
  line L370 (10.9291, 0.3981) -> (10.9291, -1.0752)
  line L371 (12.1568, -1.0752) -> (11.4517, -1.0752)
  line L372 (11.4517, -1.0752) -> (11.4517, 1.1882)
  line L373 (11.4517, 1.1882) -> (12.1568, 1.1882)
  line L374 (12.1568, 1.1882) -> (12.1568, -1.0752)
  line L375 (12.1786, 1.5115) -> (11.4323, 1.5115)
  line L376 (11.4323, 1.5115) -> (11.4323, 2.061)
  line L377 (11.4323, 2.061) -> (12.1786, 2.061)
  line L378 (12.1786, 2.061) -> (12.1786, 1.5115)
  spline S238 degree 2 poles (13.9436, -0.8345) (13.8707, -0.8953) (13.7564, -0.9925) (13.6592, -1.0411) knots 0 0 0 1 2 2 2
  spline S239 degree 2 poles (13.6592, -1.0411) (13.5644, -1.0873) (13.3845, -1.1359) (13.224, -1.1359) knots 0 0 0 1 2 2 2
  spline S240 degree 2 poles (13.224, -1.1359) (12.9226, -1.1359) (12.5263, -0.7324) (12.5263, -0.4261) knots 0 0 0 1 2 2 2
  spline S241 degree 2 poles (12.5263, -0.4261) (12.5263, -0.1757) (12.7281, 0.1355) (12.9177, 0.2255) knots 0 0 0 1 2 2 2